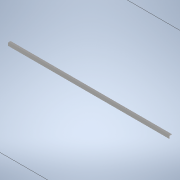
# Autodesk Inventor part: SP39V1 Chapa Acrilico
Saved by Autodesk Inventor 2021.2 (Build 252289000, 289)
## iProperties
Created: 2026-08-21
Part Number: SP39V1 Chapa Acrilico
Material: Generic
Document SubType Name: Sheet Metal
Designer: nelso
Density: 1 g/cm^3
Sheet Metal Rule: Default_mm
Appearance: Default
Author: nelso
Autodesk Inventor part; units mm, degrees
ref_plane "YZ Plane" through (0, 0, 0) normal (1, 0, 0) x (0, 1, 0)
ref_plane "XZ Plane" through (0, 0, 0) normal (0, 1, 0) x (-1, 0, 0)
ref_plane "XY Plane" through (0, 0, 0) normal (0, 0, 1) x (1, 0, 0)
sketch "Sketch1" plane through (0, 0, 0) normal (0, 1, 0) x (-1, 0, 0)
  line L0 (825, 15) -> (-825, 15)
  line L1 (-825, 15) -> (-825, -15)
  line L2 (-825, -15) -> (825, -15)
  line L3 (825, -15) -> (825, 15)
  line L4 (825, 15) -> (-825, -15) construction
  line L5 (-825, 15) -> (825, -15) construction
  point P0 (0, 0)
  dimension "d0" = 1650
  dimension "d1" = 30
  measures "d0" distance of L2.end L1.end
  measures "d1" distance of L1.end L0.end
extrude "Plate1" add sketch "Sketch1" along normal blind 3.2
sketch "Sketch2" plane through (825, 0, 11.8) normal (0, 0, 1) x (1, 0, 0)
  line L0 (-1650, 0) -> (0, 0)
  line L1 (0, 0) -> (0, 25)
  line L2 (0, 25) -> (-1650, 25)
  line L3 (-1650, 25) -> (-1650, 0)
  constraints: 6 end point, 1 horizontal, 1 perpendicular, 1 vertical
edge flange "Flange1" height 25 angle 90 thickness 3.2 bend radius 1.516 thickness toward (0, 0, 1) relief straight relief width 3.2 relief depth 1.6 edges at (0, 3.2, 15) wall of the first edge with corners at (-825, 0, 11.8) (825, 0, 11.8) (825, 25, 11.8) (-825, 25, 11.8)
bend "Bend1"
corner "Corner1"
sketch "Sketch3" plane through (825, 25, 11.8) normal (0, 0, -1) x (-1, 0, 0)
  circle A0 centre (105, -10.45) radius 1.5706 projected
  circle A1 centre (285, -10.45) radius 1.5706 projected
  circle A2 centre (465, -10.45) radius 1.5706 projected
  circle A3 centre (645, -10.45) radius 1.5706 projected
  circle A4 centre (825, -10.45) radius 1.5706 projected
  circle A5 centre (1005, -10.45) radius 1.5706 projected
  circle A6 centre (1185, -10.45) radius 1.5706 projected
  circle A7 centre (1365, -10.45) radius 1.5706 projected
  circle A8 centre (1545, -10.45) radius 1.5706 projected
  point P0 (825, -25)
hole "Hole1" at (540, 14.55, 11.8) at (720, 14.55, 11.8) at (360, 14.55, 11.8) at (180, 14.55, 11.8) at (0, 14.55, 11.8) at (-180, 14.55, 11.8) at (-360, 14.55, 11.8) at (-540, 14.55, 11.8) at (-720, 14.55, 11.8) direction (0, 0, 1) diameter 4.5 depth 3.2 tip angle 118 clearance for "Countersunk Flat Head Screw ISO 2009/7046" size "M4" standard "ISO"
equation "\"d18\" = Thickness"
equation "\"d2\" = Thickness"
equation "\"d3\" = BendReliefWidth"
equation "\"d4\" = BendReliefDepth"
equation "\"d5\" = MinimumRemnant"
equation "\"d6\" = TransitionRadius"
equation "\"d9\" = BendRadius"
equation "\"d10\" = CornerReliefSize"
equation "\"d11\" = GapSize"
equation "\"d12\" = JacobiRadiusSize"
equation "\"BendReliefWidth\" = Thickness"
equation "\"BendReliefDepth\" = 0.5 * Thickness"
equation "\"CornerReliefSize\" = 4 * Thickness"
equation "\"MinimumRemnant\" = 2 * Thickness"
equation "\"TransitionRadius\" = BendRadius"
equation "\"JacobiRadiusSize\" = BendRadius"
equation "\"GapSize\" = Thickness"
equation "\"Thickness\" = 3.2"
equation "\"BendRadius\" = 1.516"
body "Solid1"
